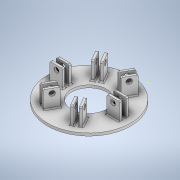
# Autodesk Inventor part: inner_hub
Saved by Autodesk Inventor 2020 (Build 240168000, 168)
## iProperties
Created: 2019-09-17
Part Number: inner_hub
Material: Generic
Document SubType Name: Modeling
Designer: dlr6513
Density: 1 g/cm^3
Appearance: Default
Author: dlr6513
Autodesk Inventor part; units mm, degrees
ref_plane "YZ Plane" through (0, 0, 0) normal (1, 0, 0) x (0, 1, 0)
ref_plane "XZ Plane" through (0, 0, 0) normal (0, 1, 0) x (-1, 0, 0)
ref_plane "XY Plane" through (0, 0, 0) normal (0, 0, 1) x (1, 0, 0)
sketch "Sketch1" plane through (0, 0, 0) normal (0, 1, 0) x (-1, 0, 0)
  circle A0 centre (17.7898, 49.4826) radius 40
  circle A1 centre (17.7898, 49.4826) radius 20
  point P0 (0, 0)
  dimension "d0" = 80
  dimension "d1" = 40
  constraints: 2 centre point, 1 coincident
  measures "d0" diameter of A0
  measures "d1" diameter of A1
extrude "Extrusion1" add sketch "Sketch1" along normal blind 3
sketch "Sketch2" plane through (-17.7898, 3, 49.4826) normal (0, 1, 0) x (1, 0, 0)
  point P0 (17.7898, 49.4826)
sketch "Sketch3" plane through (-17.7898, 3, 49.4826) normal (0, 1, 0) x (1, 0, 0)
  circle A0 centre (0, 0) radius 40 projected
  line L0 (-25.4376, 2.5) -> (-25.4376, 5)
  line L1 (-25.4376, 5) -> (-39.6863, 5)
  line L2 (-25.4376, -2.5) -> (-25.4376, -5)
  line L3 (-25.4376, -5) -> (-39.6863, -5)
  line L4 (-39.9218, 2.5) -> (-25.4376, 2.5)
  line L5 (-39.9218, -2.5) -> (-25.4376, -2.5)
  line L6 (-8.3887, -24.5296) -> (-15.513, -36.8693)
  line L7 (-17.7958, -35.8233) -> (-10.5537, -23.2796)
  line L8 (-10.5537, -23.2796) -> (-8.3887, -24.5296)
  line L9 (-14.8839, -20.7796) -> (-17.0489, -19.5296)
  line L10 (-17.0489, -19.5296) -> (-24.1733, -31.8693)
  line L11 (-22.126, -33.3233) -> (-14.8839, -20.7796)
  line L12 (17.0489, -19.5296) -> (24.1733, -31.8693)
  line L13 (22.126, -33.3233) -> (14.8839, -20.7796)
  line L14 (14.8839, -20.7796) -> (17.0489, -19.5296)
  line L15 (10.5537, -23.2796) -> (8.3887, -24.5296)
  line L16 (8.3887, -24.5296) -> (15.513, -36.8693)
  line L17 (17.7958, -35.8233) -> (10.5537, -23.2796)
  line L18 (25.4376, 5) -> (39.6863, 5)
  line L19 (39.9218, 2.5) -> (25.4376, 2.5)
  line L20 (25.4376, 2.5) -> (25.4376, 5)
  line L21 (25.4376, -2.5) -> (25.4376, -5)
  line L22 (25.4376, -5) -> (39.6863, -5)
  line L23 (39.9218, -2.5) -> (25.4376, -2.5)
  line L24 (8.3887, 24.5296) -> (15.513, 36.8693)
  line L25 (17.7958, 35.8233) -> (10.5537, 23.2796)
  line L26 (10.5537, 23.2796) -> (8.3887, 24.5296)
  line L27 (14.8839, 20.7796) -> (17.0489, 19.5296)
  line L28 (17.0489, 19.5296) -> (24.1733, 31.8693)
  line L29 (22.126, 33.3233) -> (14.8839, 20.7796)
  line L30 (-17.0489, 19.5296) -> (-24.1733, 31.8693)
  line L31 (-22.126, 33.3233) -> (-14.8839, 20.7796)
  line L32 (-14.8839, 20.7796) -> (-17.0489, 19.5296)
  line L33 (-10.5537, 23.2796) -> (-8.3887, 24.5296)
  line L34 (-8.3887, 24.5296) -> (-15.513, 36.8693)
  line L35 (-17.7958, 35.8233) -> (-10.5537, 23.2796)
  point P0 (17.7898, 49.4826)
  point P1 (-24.1733, -31.8693)
  point P2 (-22.126, -33.3233)
  point P3 (-17.7958, -35.8233)
  point P4 (-15.513, -36.8693)
  point P5 (17.7958, -35.8233)
  point P6 (22.126, -33.3233)
  point P7 (39.6863, -5)
  point P8 (39.9218, -2.5)
  point P9 (39.9218, 2.5)
  point P10 (39.6863, 5)
  point P11 (-24.1733, 31.8693)
  dimension "d8" = 360
  constraints: 72 end point, 4 point on circle, 85 other
extrude "Extrusion2" add sketch "Sketch3" along normal blind 20 contours L19 L20 L18 A0 | A0 L22 L21 L23 | L28 L27 L29 A0 | A0 L13 L14 L12 | L25 L26 L24 A0 | A0 L16 L15 L17 | L34 L33 L35 A0 | A0 L7 L8 L6 | L31 L32 L30 A0 | A0 L10 L9 L11 | L1 L0 L4 A0 | A0 L5 L2 L3
sketch "Sketch4" plane through (21.8964, 3, 44.4826) normal (0, 0, -1) x (-1, 0, 0)
  point P0 (21.8964, -3)
sketch "Sketch5" plane through (-0.7409, 3, 69.0122) normal (0.8660254, 0, -0.5) x (-0.5, 0, -0.8660254)
  circle A0 centre (-6.7487, 15) radius 2.5
  line L0 (-14.2487, 20) -> (0, 20) projected
  line L1 (-14.2487, 0) -> (-14.2487, 20) projected
  point P0 (59.3959, -3)
  dimension "d12" = 5
  dimension "d13" = 5
  dimension "d14" = 7.5
  constraints: 1 centre point
  measures "d12" diameter of A0
  measures "d13" distance from line of L0 A0.centre
  measures "d14" distance from line of L1 A0.centre
extrude "Extrusion3" cut sketch "Sketch5" against normal through all
sketch "Sketch6" plane through (-26.1785, 3, 74.0122) normal (0.8660254, 0, 0.5) x (0.5, 0, -0.8660254)
  circle A0 centre (-6.7487, 15) radius 2.5
  line L0 (-14.2487, 20) -> (0, 20) projected
  line L1 (-14.2487, 0) -> (-14.2487, 20) projected
  point P0 (77.1857, -3)
  dimension "d17" = 5
  dimension "d18" = 5
  dimension "d19" = 7.5
  constraints: 1 centre point
  measures "d17" diameter of A0
  measures "d18" distance from line of L0 A0.centre
  measures "d19" distance from line of L1 A0.centre
extrude "Extrusion4" cut sketch "Sketch6" against normal through all
sketch "Sketch7" plane through (-57.4761, 3, 54.4826) normal (0, 0, 1) x (1, 0, 0)
  circle A0 centre (7.5, 15) radius 2.5
  line L0 (0, 20) -> (14.2487, 20) projected
  line L1 (0, 0) -> (0, 20) projected
  point P0 (57.4761, -3)
  dimension "d22" = 5
  dimension "d23" = 5
  dimension "d24" = 7.5
  constraints: 1 centre point
  measures "d22" diameter of A0
  measures "d23" distance from line of L0 A0.centre
  measures "d24" distance from line of L1 A0.centre
extrude "Extrusion5" cut sketch "Sketch7" against normal through all
sketch "Sketch8" plane through (-34.8388, 3, 29.953) normal (-0.8660254, 0, 0.5) x (0.5, 0, 0.8660254)
  circle A0 centre (-6.7487, 15) radius 2.5
  line L0 (-14.2487, 20) -> (0, 20) projected
  line L1 (-14.2487, 0) -> (-14.2487, 20) projected
  point P0 (-8.5207, -3)
  dimension "d27" = 5
  dimension "d28" = 5
  dimension "d29" = 7.5
  constraints: 1 centre point
  measures "d27" diameter of A0
  measures "d28" distance from line of L0 A0.centre
  measures "d29" distance from line of L1 A0.centre
extrude "Extrusion6" cut sketch "Sketch8" against normal through all
sketch "Sketch9" plane through (21.8964, 3, 44.4826) normal (0, 0, -1) x (-1, 0, 0)
  circle A0 centre (7.5, 15) radius 2.5
  line L0 (0, 20) -> (14.2487, 20) projected
  line L1 (0, 0) -> (0, 20) projected
  point P0 (21.8964, -3)
  dimension "d32" = 5
  dimension "d33" = 5
  dimension "d34" = 7.5
  constraints: 1 centre point
  measures "d32" diameter of A0
  measures "d33" distance from line of L0 A0.centre
  measures "d34" distance from line of L1 A0.centre
extrude "Extrusion7" cut sketch "Sketch9" against normal through all
sketch "Sketch10" plane through (-9.4011, 3, 24.953) normal (-0.8660254, 0, -0.5) x (-0.5, 0, 0.8660254)
  circle A0 centre (-6.7487, 15) radius 2.5
  line L0 (-14.2487, 20) -> (0, 20) projected
  line L1 (-14.2487, 0) -> (-14.2487, 20) projected
  point P0 (-26.3105, -3)
  dimension "d37" = 5
  dimension "d38" = 5
  dimension "d39" = 7.5
  constraints: 1 centre point
  measures "d37" diameter of A0
  measures "d38" distance from line of L0 A0.centre
  measures "d39" distance from line of L1 A0.centre
extrude "Extrusion8" cut sketch "Sketch10" against normal through all
fillet "Fillet1" radius 1.27 12 edges at (-1.8234, 3, 69.6372) (-8.3186, 3, 73.3872) (-27.261, 3, 73.3872) (-33.7562, 3, 69.6372) (-43.2274, 3, 53.2326) (-43.2274, 3, 45.7326) (-27.261, 3, 25.578) (-33.7562, 3, 29.328) (-8.3186, 3, 25.578) (-1.8234, 3, 29.328) (7.6478, 3, 45.7326) (7.6478, 3, 53.2326)
fillet "Fillet2" radius 1.27 24 edges at (-8.3186, 23, 25.578) (-1.8234, 23, 29.328) (-1.1272, 23, 13.1184) (5.3712, 23, 16.8702) (22.0338, 23, 45.7308) (7.6478, 23, 45.7326) (7.6478, 23, 53.2326) (22.0338, 23, 53.2345) (-8.3186, 23, 73.3872) (-1.8234, 23, 69.6372) (5.3712, 23, 82.095) (-1.1272, 23, 85.8468) (-34.4525, 23, 85.8468) (-40.9508, 23, 82.095) (-27.261, 23, 73.3872) (-33.7562, 23, 69.6372) (-43.2274, 23, 53.2326) (-43.2274, 23, 45.7326) (-57.6135, 23, 53.2345) (-57.6135, 23, 45.7308) (-40.9508, 23, 16.8702) (-34.4525, 23, 13.1184) (-27.261, 23, 25.578) (-33.7562, 23, 29.328)
fillet "Fillet3" radius 0.381 24 edges at (-52.4761, 18, 54.4826) (-52.4761, 18, 51.9826) (-52.4761, 18, 44.4826) (-52.4761, 18, 46.9826) (-39.4631, 18, 21.9434) (-37.298, 18, 20.6934) (-30.8028, 18, 16.9434) (-32.9679, 18, 18.1934) (-4.7768, 18, 16.9434) (-2.6118, 18, 18.1934) (3.8834, 18, 21.9434) (1.7184, 18, 20.6934) (16.8964, 18, 54.4826) (16.8964, 18, 51.9826) (16.8964, 18, 44.4826) (16.8964, 18, 46.9826) (3.8834, 18, 77.0218) (1.7184, 18, 78.2718) (-4.7768, 18, 82.0218) (-2.6118, 18, 80.7718) (-39.4631, 18, 77.0218) (-37.298, 18, 78.2718) (-30.8028, 18, 82.0218) (-32.9679, 18, 80.7718)
fillet "Fillet4" radius 1.27 48 edges at (-34.5213, 3, 68.4623) (-38.4009, 3, 75.1821) (-36.2947, 3, 76.5341) (-32.3562, 3, 69.7123) (-28.0261, 3, 72.2123) (-31.9646, 3, 79.0341) (-29.7407, 3, 80.1821) (-25.861, 3, 73.4623) (-50.3518, 3, 54.4826) (-42.5924, 3, 54.4826) (-42.5924, 3, 51.9826) (-50.4695, 3, 51.9826) (-42.5924, 3, 44.4826) (-50.3518, 3, 44.4826) (-50.4695, 3, 46.9826) (-42.5924, 3, 46.9826) (-34.5213, 3, 30.5029) (-38.4009, 3, 23.7832) (-36.2947, 3, 22.4312) (-32.3562, 3, 29.2529) (-29.7407, 3, 18.7832) (-25.861, 3, 25.5029) (-28.0261, 3, 26.7529) (-31.9646, 3, 19.9312) (-9.7186, 3, 25.5029) (-5.839, 3, 18.7832) (-3.615, 3, 19.9312) (-7.5536, 3, 26.7529) (2.8213, 3, 23.7832) (-1.0584, 3, 30.5029) (-3.2235, 3, 29.2529) (0.7151, 3, 22.4312) (7.0128, 3, 44.4826) (14.7721, 3, 44.4826) (14.8899, 3, 46.9826) (7.0128, 3, 46.9826) (14.7721, 3, 54.4826) (7.0128, 3, 54.4826) (7.0128, 3, 51.9826) (14.8899, 3, 51.9826) (-1.0584, 3, 68.4623) (2.8213, 3, 75.1821) (-3.615, 3, 79.0341) (-7.5536, 3, 72.2123) (-3.2235, 3, 69.7123) (0.7151, 3, 76.5341) (-9.7186, 3, 73.4623) (-5.839, 3, 80.1821)
sketch "Sketch11" plane through (0, 3, 0) normal (0, 1, 0) x (1, 0, 0)
  circle A0 centre (-17.7898, -49.4826) radius 40 projected
  circle A1 centre (-17.7898, -49.4826) radius 47.3921
  point P0 (0, 0)
  constraints: 1 centre point, 1 coincident
extrude "Extrusion9" add sketch "Sketch11" against normal blind 3
body "Solid1"
